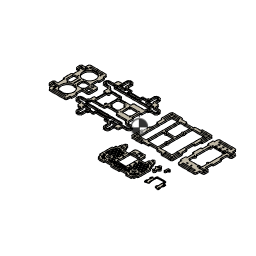
v109 (Autodesk Fusion 360 design; units mm, degrees)
Autodesk Fusion 360 part; units mm, degrees
note: some values were not read from the file. Set by a fixed rule: which sketch regions a step uses.
(part 1 of 3)
sketch "Schizzo1" plane through (0, 0, 0) normal (0, 1, 0) x (1, 0, 0)
  line L0 (-131, 140) -> (-131, 145)
  line L1 (-131, 145) -> (-111, 145)
  line L2 (-111, 140) -> (-131, 140)
  line L3 (-111, 145) -> (-111, 140)
  line L4 (-86, 145) -> (-86, 140)
  line L5 (-86, 140) -> (-71, 140)
  line L6 (-106, 147) -> (-106, 148)
  line L7 (-141, 150) -> (-108, 150)
  arc A0 (-106, 147) -> (-104, 145) centre (-104, 147) ccw
  arc A1 (-106, 148) -> (-108, 150) centre (-108, 148) ccw
  line L8 (25, 10) -> (25, 5)
  line L9 (30, 0) -> (57.5, 0)
  arc A2 (25, 5) -> (30, 0) centre (30, 5) ccw
  arc A3 (-141, 150) -> (-146, 145) centre (-141, 145) ccw
  line L10 (25, 15) -> (20, 15)
  line L11 (20, 35) -> (25, 35)
  line L12 (25, 60) -> (20, 60)
  line L13 (20, 60) -> (20, 75)
  line L14 (25, 10) -> (25, 15)
  line L15 (25, 35) -> (25, 60)
  line L16 (-141, 90) -> (-136, 90)
  line L17 (-136, 90) -> (-136, 75)
  line L18 (-143, 110) -> (-144, 110)
  line L19 (-146, 112) -> (-146, 145)
  arc A4 (-146, 112) -> (-144, 110) centre (-144, 112) ccw
  arc A5 (-141, 108) -> (-143, 110) centre (-143, 108) ccw
  line L20 (-141, 115) -> (-136, 115)
  line L21 (-136, 115) -> (-136, 135)
  line L22 (-136, 135) -> (-141, 135)
  line L23 (-141, 135) -> (-141, 115)
  arc A6 (-108, 0) -> (-106, 2) centre (-108, 2) ccw
  line L24 (-106, 3) -> (-106, 2)
  arc A7 (-104, 5) -> (-106, 3) centre (-104, 3) ccw
  line L25 (-86, 5) -> (-86, 10)
  line L26 (-86, 10) -> (-71, 10)
  line L27 (-136, 60) -> (-136, 75)
  line L28 (-141, 60) -> (-136, 60)
  arc A8 (-143, 40) -> (-141, 42) centre (-143, 42) ccw
  line L29 (-143, 40) -> (-144, 40)
  arc A9 (-144, 40) -> (-146, 38) centre (-144, 38) ccw
  line L30 (-146, 38) -> (-146, 5)
  arc A10 (-146, 5) -> (-141, 0) centre (-141, 5) ccw
  line L31 (-141, 0) -> (-108, 0)
  line L32 (-111, 10) -> (-131, 10)
  line L33 (-131, 10) -> (-131, 5)
  line L34 (-111, 5) -> (-111, 10)
  line L35 (-131, 5) -> (-111, 5)
  line L36 (-141, 15) -> (-141, 35)
  line L37 (-141, 35) -> (-136, 35)
  line L38 (-136, 15) -> (-141, 15)
  line L39 (-136, 35) -> (-136, 15)
  arc A11 (1, 110) -> (-1, 108) centre (1, 108) ccw
  line L40 (1, 110) -> (2, 110)
  arc A12 (2, 110) -> (4, 112) centre (2, 112) ccw
  line L41 (4, 112) -> (4, 145)
  arc A13 (4, 145) -> (-1, 150) centre (-1, 145) ccw
  line L42 (-1, 150) -> (-34, 150)
  arc A14 (-34, 150) -> (-36, 148) centre (-34, 148) ccw
  line L43 (-36, 147) -> (-36, 148)
  arc A15 (-38, 145) -> (-36, 147) centre (-38, 147) ccw
  line L44 (-56, 145) -> (-56, 140)
  line L45 (-56, 140) -> (-71, 140)
  line L46 (-31, 140) -> (-11, 140)
  line L47 (-11, 140) -> (-11, 145)
  line L48 (-31, 145) -> (-31, 140)
  line L49 (-11, 145) -> (-31, 145)
  line L50 (-1, 135) -> (-1, 115)
  line L51 (-1, 115) -> (-6, 115)
  line L52 (-6, 135) -> (-1, 135)
  line L53 (-6, 115) -> (-6, 135)
  line L54 (-1, 90) -> (-6, 90)
  line L55 (-6, 90) -> (-6, 75)
  line L56 (-1, 60) -> (-6, 60)
  line L57 (-6, 60) -> (-6, 75)
  line L58 (-56, 5) -> (-56, 10)
  line L59 (-56, 10) -> (-71, 10)
  arc A16 (-1, 42) -> (1, 40) centre (1, 42) ccw
  line L60 (1, 40) -> (2, 40)
  arc A17 (4, 38) -> (2, 40) centre (2, 38) ccw
  line L61 (4, 38) -> (4, 5)
  arc A18 (-1, 0) -> (4, 5) centre (-1, 5) ccw
  line L62 (-1, 0) -> (-34, 0)
  arc A19 (-36, 2) -> (-34, 0) centre (-34, 2) ccw
  line L63 (-36, 3) -> (-36, 2)
  arc A20 (-36, 3) -> (-38, 5) centre (-38, 3) ccw
  line L64 (-11, 10) -> (-11, 5)
  line L65 (-11, 5) -> (-31, 5)
  line L66 (-31, 10) -> (-11, 10)
  line L67 (-31, 5) -> (-31, 10)
  line L68 (-1, 15) -> (-1, 35)
  line L69 (-1, 35) -> (-6, 35)
  line L70 (-6, 15) -> (-1, 15)
  line L71 (-6, 35) -> (-6, 15)
  line L72 (-231.9997, 2.9999) -> (-231.9997, 2.0006)
  line L73 (-192, 38) -> (-192, 37.0001)
  line L74 (-307, 5) -> (-307, 10)
  line L75 (-197, 60) -> (-202, 60)
  arc A21 (-300, 5) -> (-302, 3) centre (-300, 3) ccw
  arc A22 (-304, 0) -> (-302, 2) centre (-304, 2) ccw
  arc A23 (-197, -0.0001) -> (-192, 4.9999) centre (-197, 4.9999) ccw
  arc A24 (-197, 42) -> (-195, 40) centre (-195, 42) ccw
  arc A25 (-342.0001, 5) -> (-337, 0) centre (-337, 5) ccw
  line L76 (-302, 3) -> (-302, 2)
  line L77 (-195, 40) -> (-194, 40)
  arc A26 (-340, 40) -> (-342, 38) centre (-340, 38) ccw
  arc A27 (-192, 38) -> (-194, 40) centre (-194, 38) ccw
  line L78 (-339, 40) -> (-340, 40)
  line L79 (-202, 60) -> (-202, 75)
  arc A28 (-339, 40) -> (-337, 42) centre (-339, 42) ccw
  arc A29 (-231.9997, 2.9999) -> (-233.9999, 5.0001) centre (-233.9999, 2.9999) ccw
  arc A30 (-231.9997, 2.0006) -> (-229.999, -0.0001) centre (-229.999, 2.0006) ccw
  line L80 (85, 0) -> (57.5, 0)
  arc A31 (85, 0) -> (90, 5) centre (85, 5) ccw
  line L81 (90, 35) -> (90, 60)
  line L82 (90, 60) -> (95, 60)
  line L83 (95, 60) -> (95, 75)
  line L84 (20, 115) -> (25, 115)
  line L85 (25, 115) -> (25, 90)
  line L86 (25, 90) -> (20, 90)
  line L87 (20, 90) -> (20, 75)
  line L88 (25, 140) -> (25, 145)
  line L89 (30, 150) -> (57.5, 150)
  arc A32 (30, 150) -> (25, 145) centre (30, 145) ccw
  line L90 (25, 135) -> (20, 135)
  line L91 (25, 140) -> (25, 135)
  line L92 (57.5, 140) -> (35, 140)
  line L93 (35, 145) -> (35, 140)
  line L94 (57.5, 145) -> (35, 145)
  line L95 (80, 145) -> (80, 140)
  line L96 (80, 140) -> (57.5, 140)
  line L97 (57.5, 145) -> (80, 145)
  arc A33 (90, 145) -> (85, 150) centre (85, 145) ccw
  line L98 (85, 150) -> (57.5, 150)
  line L99 (90, 90) -> (95, 90)
  line L100 (95, 90) -> (95, 75)
  line L101 (-452, 90) -> (-452, 75)
  line L102 (-452, 60) -> (-452, 75)
  line L103 (-452, 115) -> (-457, 115)
  line L104 (-437, 5) -> (-437, 10)
  line L105 (-382, 35) -> (-382, 57.5)
  line L106 (-442, 150) -> (-414.5, 150)
  line L107 (-357, 62.5) -> (-357, 75)
  line L108 (-447, 140) -> (-447, 145)
  line L109 (-377, 115) -> (-382, 115)
  line L110 (-357, 87.5) -> (-357, 75)
  line L111 (-447, 35) -> (-447, 60)
  arc A34 (-442, 150) -> (-447, 145) centre (-442, 145) ccw
  line L112 (-382, 92.5) -> (-362, 92.5)
  line L113 (-382, 140) -> (-382, 135)
  line L114 (-447, 115) -> (-447, 90)
  line L115 (-382, 135) -> (-377, 135)
  line L116 (-382, 140) -> (-382, 145)
  line L117 (-452, 115) -> (-447, 115)
  line L118 (-382, 10) -> (-382, 5)
  line L119 (-392, 5) -> (-392, 10)
  line L120 (-457, 115) -> (-457, 115)
  line L121 (-462, 130) -> (-462, 120)
  arc A35 (-462, 120) -> (-457, 115) centre (-457, 120) ccw
  arc A36 (-457, 135) -> (-462, 130) centre (-457, 130) ccw
  line L122 (-414.5, 5) -> (-437, 5)
  arc A37 (-382, 145) -> (-387, 150) centre (-387, 145) ccw
  line L123 (-447, 10) -> (-447, 5)
  line L124 (-382, 10) -> (-382, 15)
  line L125 (-447, 140) -> (-447, 135)
  line L126 (-382, 115) -> (-382, 92.5)
  line L127 (-387, 0) -> (-414.5, 0)
  line L128 (-377, 35) -> (-382, 35)
  line L129 (-447, 10) -> (-447, 15)
  line L130 (-387, 150) -> (-414.5, 150)
  line L131 (-382, 57.5) -> (-362, 57.5)
  arc A38 (-387, 0) -> (-382, 5) centre (-387, 5) ccw
  line L132 (-414.5, 5) -> (-392, 5)
  line L133 (-442, 0) -> (-414.5, 0)
  line L134 (-382, 15) -> (-377, 15)
  line L135 (-447, 90) -> (-452, 90)
  line L136 (-447, 60) -> (-452, 60)
  arc A39 (-447, 5) -> (-442, 0) centre (-442, 5) ccw
  arc A40 (-357, 87.5) -> (-362, 92.5) centre (-362, 87.5) ccw
  arc A41 (-362, 57.5) -> (-357, 62.5) centre (-362, 62.5) ccw
  circle A42 centre (-252.9, 89.1) radius 1.25
  circle A43 centre (-281.1, 60.9) radius 1.25
  line L137 (-252.9, 84.1) -> (-250.5, 84.1)
  line L138 (-257.9, 89.1) -> (-257.9, 91.5)
  line L139 (-281.1, 65.9) -> (-283.5, 65.9)
  line L140 (-276.1, 60.9) -> (-276.1, 58.5)
  arc A44 (-257.9, 89.1) -> (-252.9, 84.1) centre (-252.9, 89.1) ccw
  arc A45 (-276.1, 60.9) -> (-281.1, 65.9) centre (-281.1, 60.9) ccw
  arc A46 (-248, 81.6) -> (-250.5, 84.1) centre (-250.5, 81.6) ccw
  arc A47 (-257.9, 91.5) -> (-260.4, 94) centre (-260.4, 91.5) ccw
  arc A48 (-286, 68.4) -> (-283.5, 65.9) centre (-283.5, 68.4) ccw
  arc A49 (-276.1, 58.5) -> (-273.6, 56) centre (-273.6, 58.5) ccw
  line L141 (-31, 140) -> (-25, 140)
  line L142 (-337, 42) -> (-337, 57.5)
  line L143 (-300, 5) -> (-286.5, 5)
  line L144 (-247.5, 5.0001) -> (-233.9999, 5.0001)
  circle A50 centre (33, 54) radius 1.5
  circle A51 centre (33, 112) radius 1.5
  circle A52 centre (-115.5198, -118.5231) radius 1.5
  circle A53 centre (-134.2581, -99.7848) radius 1.5
  circle A54 centre (-120.8585, -105.1234) radius 6
  circle A55 centre (-98.9028, -64.4294) radius 1.5
  line L145 (-82.3205, -124) -> (-80, -124)
  line L146 (-85, -121) -> (-85, -122)
  line L147 (-132, -119) -> (-133, -119)
  line L148 (-135, -117) -> (-135, -116)
  line L149 (-130, -61) -> (-130, -62)
  line L150 (-120, -62) -> (-120, -61)
  line L151 (-80, -124) -> (-77.6795, -124)
  line L152 (-75, -114) -> (-79.3301, -116.5)
  line L153 (-79.3301, -116.5) -> (-79.3301, -121.5)
  line L154 (-79.3301, -121.5) -> (-75, -124)
  arc A56 (-85, -121) -> (-87, -119) centre (-87, -121) ccw
  arc A57 (-85, -122) -> (-84.2458, -123.5646) centre (-83, -122) ccw
  arc A58 (-135, -117) -> (-133, -119) centre (-133, -117) ccw
  arc A59 (-135, -116) -> (-135.7542, -114.4354) centre (-137, -116) ccw
  arc A60 (-130.6699, -119.5064) -> (-132, -119) centre (-132, -121) ccw
  arc A61 (-128, -59) -> (-130, -61) centre (-128, -61) ccw
  arc A62 (-120, -61) -> (-122, -59) centre (-122, -61) ccw
  arc A63 (-103.7753, -65.5513) -> (-105.7243, -64) centre (-105.7243, -66) ccw
  line L155 (-75, -114) -> (-79.3301, -116.5)
  line L156 (-79.3301, -116.5) -> (-79.3301, -121.5)
  line L157 (-79.3301, -121.5) -> (-75, -124)
  arc A64 (-120.6699, -117.2162) -> (-122.2488, -116.0352) centre (-122.5016, -118.0192) ccw
  arc A65 (-130.5673, -96.4116) -> (-127.8245, -96.6102) centre (-129.091, -95.0624) ccw
  arc A66 (-112.3453, -112.0894) -> (-112.7588, -113.747) centre (-110.7974, -113.356) ccw
  line L158 (-84.2458, -123.5646) -> (-80.6699, -121.5)
  line L159 (-80.6699, -121.5) -> (-80.6699, -116.5)
  line L160 (-80.6699, -116.5) -> (-85, -114)
  line L161 (-85, -114) -> (-89.3301, -116.5)
  line L162 (-89.3301, -116.5) -> (-89.3301, -119)
  line L163 (-90.6699, -119) -> (-90.6699, -116.5)
  line L164 (-90.6699, -116.5) -> (-95, -114)
  line L165 (-95, -114) -> (-99.3301, -116.5)
  line L166 (-99.3301, -116.5) -> (-99.3301, -119)
  line L167 (-126.72, -114.993) -> (-129.3301, -116.5)
  line L168 (-129.3301, -116.5) -> (-129.3301, -121.5)
  line L169 (-129.3301, -121.5) -> (-125, -124)
  line L170 (-125, -124) -> (-120.6699, -121.5)
  line L171 (-120.6699, -121.5) -> (-120.6699, -117.2162)
  line L172 (-130.6699, -116.5) -> (-135, -114)
  line L173 (-80, -115.3397) -> (-75.6699, -112.8397)
  line L174 (-75.6699, -112.8397) -> (-75.6699, -107.8397)
  line L175 (-75.6699, -107.8397) -> (-77.9904, -106.5)
  line L176 (-82.0096, -106.5) -> (-84.3301, -107.8398)
  line L177 (-84.3301, -107.8398) -> (-84.3301, -112.8398)
  line L178 (-84.3301, -112.8398) -> (-80, -115.3397)
  line L179 (-85.6699, -112.8397) -> (-85.6699, -107.8397)
  line L180 (-85.6699, -107.8397) -> (-87.9002, -106.5521)
  line L181 (-92.1651, -106.5898) -> (-94.3301, -107.8398)
  line L182 (-94.3301, -107.8398) -> (-94.3301, -112.8398)
  line L183 (-94.3301, -112.8398) -> (-90, -115.3397)
  line L184 (-90, -115.3397) -> (-85.6699, -112.8397)
  line L185 (-75.6699, -112.8397) -> (-75.6699, -107.8397)
  line L186 (-75.6699, -107.8397) -> (-77.9904, -106.5)
  line L187 (-82.0096, -106.5) -> (-84.3301, -107.8398)
  line L188 (-84.3301, -107.8398) -> (-84.3301, -112.8398)
  line L189 (-84.3301, -112.8398) -> (-80, -115.3397)
  line L190 (-80, -115.3397) -> (-75.6699, -112.8397)
  line L191 (-105.6699, -107.8397) -> (-109.8624, -105.4192)
  line L192 (-112.7588, -113.747) -> (-110, -115.3397)
  line L193 (-110, -115.3397) -> (-105.6699, -112.8397)
  line L194 (-105.6699, -112.8397) -> (-105.6699, -107.8397)
  line L195 (-100, -115.3397) -> (-95.6699, -112.8397)
  line L196 (-95.6699, -112.8397) -> (-95.6699, -107.8397)
  line L197 (-95.6699, -107.8397) -> (-100, -105.3397)
  line L198 (-100, -105.3397) -> (-104.3301, -107.8398)
  line L199 (-104.3301, -112.8398) -> (-100, -115.3397)
  line L200 (-104.3301, -107.8398) -> (-104.3301, -112.8398)
  line L201 (-130, -115.3397) -> (-127.4968, -113.8945)
  line L202 (-131.7929, -106.3749) -> (-134.3301, -107.8398)
  line L203 (-134.3301, -112.8398) -> (-130, -115.3397)
  line L204 (-134.3301, -107.8398) -> (-134.3301, -112.8398)
  line L205 (-80, -122.6603) -> (-82.3205, -124)
  line L206 (-77.6795, -124) -> (-80, -122.6603)
  line L207 (-100.6699, -99.1795) -> (-105, -96.6795)
  line L208 (-105, -96.6795) -> (-109.3301, -99.1795)
  line L209 (-109.3301, -99.1795) -> (-109.3301, -104.1795)
  line L210 (-109.3301, -104.1795) -> (-105, -106.6795)
  line L211 (-100.6699, -104.1795) -> (-100.6699, -99.1795)
  line L212 (-105, -106.6795) -> (-100.6699, -104.1795)
  line L213 (-135, -106.6795) -> (-132.4803, -105.2248)
  line L214 (-139.3301, -103) -> (-139.3301, -104.1795)
  line L215 (-139.3301, -104.1795) -> (-135, -106.6795)
  line L216 (-105.6699, -90.5192) -> (-110, -88.0192)
  line L217 (-110, -88.0192) -> (-114.3301, -90.5192)
  line L218 (-114.3301, -90.5192) -> (-114.3301, -95.5192)
  line L219 (-114.3301, -95.5192) -> (-110, -98.0192)
  line L220 (-110, -98.0192) -> (-105.6699, -95.5192)
  line L221 (-105.6699, -95.5192) -> (-105.6699, -90.5192)
  line L222 (-125.6699, -90.5192) -> (-130, -88.0192)
  line L223 (-130, -88.0192) -> (-134.3301, -90.5192)
  line L224 (-134.3301, -90.5192) -> (-134.3301, -94.7853)
  line L225 (-125.6699, -95.2315) -> (-125.6699, -90.5192)
  line L226 (-115.6699, -95.424) -> (-115.6699, -90.5192)
  line L227 (-115.6699, -90.5192) -> (-120, -88.0192)
  line L228 (-120, -88.0192) -> (-124.3301, -90.5192)
  line L229 (-124.3301, -90.5192) -> (-124.3301, -94.6856)
  line L230 (-140, -98.0192) -> (-138.5149, -97.1618)
  line L231 (-135.6699, -94.9882) -> (-135.6699, -90.5192)
  line L232 (-135.6699, -90.5192) -> (-140, -88.0192)
  line L233 (-100.6699, -81.859) -> (-105, -79.359)
  line L234 (-105, -79.359) -> (-109.3301, -81.859)
  line L235 (-109.3301, -81.859) -> (-109.3301, -86.859)
  line L236 (-109.3301, -86.859) -> (-105, -89.359)
  line L237 (-100.6699, -86.859) -> (-100.6699, -81.859)
  line L238 (-105, -89.359) -> (-100.6699, -86.859)
  line L239 (-110.6699, -86.859) -> (-110.6699, -81.859)
  line L240 (-110.6699, -81.859) -> (-115, -79.359)
  line L241 (-115, -79.359) -> (-119.3301, -81.859)
  line L242 (-119.3301, -81.859) -> (-119.3301, -86.859)
  line L243 (-119.3301, -86.859) -> (-115, -89.359)
  line L244 (-115, -89.359) -> (-110.6699, -86.859)
  line L245 (-120.6699, -81.859) -> (-125, -79.359)
  line L246 (-125, -79.359) -> (-129.3301, -81.859)
  line L247 (-129.3301, -81.859) -> (-129.3301, -86.859)
  line L248 (-129.3301, -86.859) -> (-125, -89.359)
  line L249 (-120.6699, -86.859) -> (-120.6699, -81.859)
  line L250 (-125, -89.359) -> (-120.6699, -86.859)
  line L251 (-130.6699, -86.859) -> (-130.6699, -81.859)
  line L252 (-130.6699, -81.859) -> (-135, -79.359)
  line L253 (-135, -79.359) -> (-139.3301, -81.859)
  line L254 (-139.3301, -81.859) -> (-139.3301, -86.859)
  line L255 (-139.3301, -86.859) -> (-135, -89.359)
  line L256 (-135, -89.359) -> (-130.6699, -86.859)
  line L257 (-134.3301, -73.1987) -> (-134.3301, -78.1987)
  line L258 (-134.3301, -78.1987) -> (-130, -80.6987)
  line L259 (-130, -80.6987) -> (-125.6699, -78.1987)
  line L260 (-125.6699, -78.1987) -> (-125.6699, -73.1987)
  line L261 (-125.6699, -73.1987) -> (-130, -70.6987)
  line L262 (-130, -70.6987) -> (-134.3301, -73.1987)
  line L263 (-124.3301, -78.1987) -> (-120, -80.6987)
  line L264 (-120, -80.6987) -> (-115.6699, -78.1987)
  line L265 (-115.6699, -78.1987) -> (-115.6699, -73.1987)
  line L266 (-115.6699, -73.1987) -> (-120, -70.6987)
  line L267 (-124.3301, -73.1987) -> (-124.3301, -78.1987)
  line L268 (-120, -70.6987) -> (-124.3301, -73.1987)
  line L269 (-114.3301, -78.1987) -> (-110, -80.6987)
  line L270 (-110, -80.6987) -> (-105.6699, -78.1987)
  line L271 (-105.6699, -78.1987) -> (-105.6699, -73.1987)
  line L272 (-105.6699, -73.1987) -> (-110, -70.6987)
  line L273 (-114.3301, -73.1987) -> (-114.3301, -78.1987)
  line L274 (-110, -70.6987) -> (-114.3301, -73.1987)
  line L275 (-108.3975, -64) -> (-109.3301, -64.5385)
  line L276 (-109.3301, -64.5385) -> (-109.3301, -69.5385)
  line L277 (-109.3301, -69.5385) -> (-105, -72.0385)
  line L278 (-105, -72.0385) -> (-100.6699, -69.5385)
  line L279 (-100.6699, -69.5385) -> (-100.6699, -69.1067)
  line L280 (-118.3454, -63.9699) -> (-119.3301, -64.5385)
  line L281 (-119.3301, -64.5385) -> (-119.3301, -69.5385)
  line L282 (-119.3301, -69.5385) -> (-115, -72.0385)
  line L283 (-115, -72.0385) -> (-110.6699, -69.5385)
  line L284 (-110.6699, -64.5385) -> (-111.6025, -64)
  line L285 (-110.6699, -69.5385) -> (-110.6699, -64.5385)
  line L286 (-125, -62.0385) -> (-129.3301, -64.5385)
  line L287 (-129.3301, -64.5385) -> (-129.3301, -69.5385)
  line L288 (-129.3301, -69.5385) -> (-125, -72.0385)
  line L289 (-125, -72.0385) -> (-120.6699, -69.5385)
  line L290 (-120.6699, -64.5385) -> (-125, -62.0385)
  line L291 (-120.6699, -69.5385) -> (-120.6699, -64.5385)
  line L292 (-120, -63.3782) -> (-119.6271, -63.1629)
  line L293 (-124.3301, -59) -> (-124.3301, -60.8782)
  line L294 (-124.3301, -60.8782) -> (-120, -63.3782)
  line L295 (-130.3729, -63.163) -> (-130, -63.3782)
  line L296 (-130, -63.3782) -> (-125.6699, -60.8782)
  line L297 (-125.6699, -60.8782) -> (-125.6699, -59)
  line L298 (-87, -119) -> (-89.3301, -119)
  line L299 (-90.6699, -119) -> (-99.3301, -119)
  arc A67 (-112.3453, -112.0894) -> (-109.8624, -105.4192) centre (-120.8585, -105.1234) ccw
  arc A68 (-115.6699, -95.424) -> (-124.3301, -94.6856) centre (-120.8585, -105.1234) ccw
  arc A69 (-125.6699, -95.2315) -> (-127.8245, -96.6102) centre (-120.8585, -105.1234) ccw
  arc A70 (-130.5673, -96.4116) -> (-134.3301, -94.7853) centre (-134.2581, -99.7848) ccw
  arc A71 (-135.6699, -94.9882) -> (-138.5149, -97.1618) centre (-134.2581, -99.7848) ccw
  arc A72 (-138.0873, -103) -> (-133.8982, -104.7718) centre (-134.2581, -99.7848) ccw
  arc A73 (-131.7702, -106.5138) -> (-131.7929, -106.3749) centre (-133.7542, -106.7666) ccw
  arc A74 (-132.4803, -105.2248) -> (-133.8982, -104.7718) centre (-133.7542, -106.7666) ccw
  line L300 (-140, -88.0192) -> (-140, -98.0192)
  arc A75 (-130.3729, -63.163) -> (-130, -62) centre (-132, -62) ccw
  line L301 (-122, -59) -> (-124.3301, -59)
  line L302 (-125.6699, -59) -> (-128, -59)
  arc A76 (-120, -62) -> (-119.6271, -63.1629) centre (-118, -62) ccw
  arc A77 (-118.3454, -63.9699) -> (-118, -64) centre (-118, -62) ccw
  line L303 (-118, -64) -> (-111.6025, -64)
  line L304 (-108.3975, -64) -> (-105.7243, -64)
  arc A78 (-103.7753, -65.5513) -> (-100.6699, -69.1067) centre (-98.9028, -64.4294) ccw
  line L305 (-135, -114) -> (-135.7542, -114.4354)
  line L306 (-130.6699, -116.5) -> (-130.6699, -119.5064)
  line L307 (-60, -124) -> (-35, -124)
  line L308 (-60, -124) -> (-60, -129)
  line L309 (-35, -124) -> (-35, -129)
  line L310 (-15, -129) -> (-15, -124)
  line L311 (-35, -129) -> (-15, -129)
  arc A79 (-55.5, -39) -> (-60.5, -34) centre (-60.5, -39) ccw
  line L312 (-55.5, -59) -> (-55.5, -39)
  line L313 (-35, -59) -> (-55.5, -59)
  line L314 (-35, -59) -> (-35, -54)
  line L315 (-30, -54) -> (-20, -54)
  line L316 (-15, -54) -> (-15, -59)
  line L317 (-10, -59) -> (-15, -59)
  line L318 (-10, -69) -> (-5, -69)
  line L319 (-5, -69) -> (-5, -114)
  line L320 (-15, -124) -> (-10, -124)
  line L321 (-5, -114) -> (-10, -114)
  circle A80 centre (-29.1416, -105.1234) radius 6
  circle A81 centre (-34.4802, -118.5231) radius 1.5
  circle A82 centre (-15.7419, -99.7848) radius 1.5
  line L322 (-75, -114) -> (-75, -114)
  circle A83 centre (-51.0972, -64.4294) radius 1.5
  circle A84 centre (82, 54) radius 1.5
  circle A85 centre (82, 112) radius 1.5
  circle A86 centre (-91, 75) radius 1.5
  circle A87 centre (-59, 45) radius 1.5
  arc A88 (-131, 18) -> (-128, 15) centre (-128, 18) ccw
  arc A89 (-61.5, 69.5) -> (-64.5, 72.5) centre (-64.5, 69.5) ccw
  line L323 (-11, 17.5) -> (-11, 75)
  line L324 (-13.9289, 15) -> (-13.5, 15)
  arc A90 (-56.5, 17.5) -> (-54, 15) centre (-54, 17.5) ccw
  arc A91 (-13.5, 15) -> (-11, 17.5) centre (-13.5, 17.5) ccw
  circle A92 centre (-392, 15) radius 1.5
  circle A93 centre (-432, 55) radius 1.5
  line L325 (-260.4, 94) -> (-278, 94)
  line L326 (-286, 86) -> (-286, 68.4)
  line L327 (-273.6, 56) -> (-256, 56)
  line L328 (-248, 64) -> (-248, 81.6)
  arc A94 (-278, 94) -> (-286, 86) centre (-278, 86) ccw
  arc A95 (-256, 56) -> (-248, 64) centre (-256, 64) ccw
  arc A96 (-64.5, 15) -> (-61.5, 18) centre (-64.5, 18) ccw
  arc A97 (-128, 135) -> (-131, 132) centre (-128, 132) ccw
  line L329 (-100, 18) -> (-100, 69.5)
  line L330 (-105, 18) -> (-105, 132)
  line L331 (-64.5, 15) -> (-97, 15)
  line L332 (-131, 18) -> (-131, 132)
  arc A98 (-97, 72.5) -> (-100, 69.5) centre (-97, 69.5) ccw
  arc A99 (-100, 18) -> (-97, 15) centre (-97, 18) ccw
  arc A100 (-108, 15) -> (-105, 18) centre (-108, 18) ccw
  arc A101 (-105, 132) -> (-108, 135) centre (-108, 132) ccw
  circle A102 centre (-292, 55) radius 1.5
  circle A103 centre (-322, 95) radius 1.5
  line L333 (-377, 135) -> (-377, 115)
  line L334 (-377, 35) -> (-377, 15)
  line L335 (-326, 91) -> (-326, 50)
  line L336 (-322, 46) -> (-294, 46)
  line L337 (-292, 48) -> (-292, 49.3431)
  line L338 (-322, 100.6569) -> (-322, 102)
  line L339 (-288, 59) -> (-288, 100)
  line L340 (-320, 104) -> (-292, 104)
  arc A104 (-324.4, 91.8) -> (-320.6667, 98.7712) centre (-322, 95) ccw
  arc A105 (-289.6, 58.2) -> (-293.3333, 51.2288) centre (-292, 55) ccw
  arc A106 (-326, 50) -> (-322, 46) centre (-322, 50) ccw
  arc A107 (-288, 100) -> (-292, 104) centre (-292, 100) ccw
  arc A108 (-294, 46) -> (-292, 48) centre (-294, 48) ccw
  arc A109 (-320, 104) -> (-322, 102) centre (-320, 102) ccw
  arc A110 (-289.6, 58.2) -> (-288, 59) centre (-289, 59) ccw
  arc A111 (-324.4, 91.8) -> (-326, 91) centre (-325, 91) ccw
  arc A112 (-292, 49.3431) -> (-293.3333, 51.2288) centre (-294, 49.3431) ccw
  arc A113 (-322, 100.6569) -> (-320.6667, 98.7712) centre (-320, 100.6569) ccw
  line L341 (-62.5, -38.44) -> (-76.5, -38.44)
  line L342 (-76.5, -38.44) -> (-76.5, -52.44)
  line L343 (-76.5, -52.44) -> (-62.5, -52.44)
  line L344 (-62.5, -52.44) -> (-62.5, -38.44)
  line L345 (-361.44, 62.5) -> (-375.44, 62.5)
  line L346 (-375.44, 62.5) -> (-375.44, 76.5)
  line L347 (-375.44, 76.5) -> (-361.44, 76.5)
  line L348 (-361.44, 76.5) -> (-361.44, 62.5)
  line L349 (20, 15) -> (20, 35)
  line L350 (20, 115) -> (20, 135)
  line L351 (-366, 23.0002) -> (-366, 27.0001)
  line L352 (-342, 38) -> (-342, 37.0001)
  line L353 (-342, 13.0001) -> (-342.0001, 5)
  arc A114 (-344, 35.0001) -> (-342, 37.0001) centre (-344, 37.0001) ccw
  arc A115 (-342, 13.0001) -> (-344, 15.0001) centre (-344, 13.0001) ccw
  arc A116 (-358, 35.0001) -> (-366, 27.0001) centre (-358, 27.0001) ccw
  arc A117 (-366, 23.0002) -> (-358, 15.0002) centre (-358, 23.0002) ccw
  line L354 (-307, -2) -> (-307, -15.9102)
  line L355 (-315, -23.9102) -> (-319, -23.9102)
  line L356 (-327, -15.9102) -> (-327, -2)
  line L357 (-337, 0) -> (-329, 0)
  line L358 (-305, 0) -> (-304, 0)
  arc A118 (-327, -2) -> (-329, 0) centre (-329, -2) ccw
  arc A119 (-305, 0) -> (-307, -2) centre (-305, -2) ccw
  arc A120 (-327, -15.9102) -> (-319, -23.9102) centre (-319, -15.9102) ccw
  arc A121 (-315, -23.9102) -> (-307, -15.9102) centre (-315, -15.9102) ccw
  line L359 (-227, -2.0001) -> (-227, -15.9189)
  arc A122 (-227, -15.9189) -> (-219, -23.9102) centre (-219, -15.9102) ccw
  line L360 (-219, -23.9102) -> (-215, -23.9102)
  arc A123 (-215, -23.9102) -> (-207, -15.9246) centre (-215, -15.9102) ccw
  line L361 (-207, -15.9246) -> (-207, -2.0001)
  arc A124 (-205, -0.0001) -> (-207, -2.0001) centre (-205, -2.0001) ccw
  arc A125 (-227, -2.0001) -> (-229, -0.0001) centre (-229, -2.0001) ccw
  line L362 (-197, -0.0001) -> (-205, -0.0001)
  line L363 (-229, -0.0001) -> (-229.999, -0.0001)
  arc A126 (-190, 15.0001) -> (-192, 13.0001) centre (-190, 13.0001) ccw
  arc A127 (-175.9914, 15.0002) -> (-168, 23.0002) centre (-176, 23.0002) ccw
  line L364 (-168, 23.0002) -> (-168, 27.0001)
  arc A128 (-168, 27.0001) -> (-176, 35.0001) centre (-176, 27.0001) ccw
  arc A129 (-192, 37.0001) -> (-190, 35.0001) centre (-190, 37.0001) ccw
  line L365 (-192, 4.9999) -> (-192, 13.0001)
  line L366 (33, 35) -> (33, 46.5838)
  line L367 (33, 61.4162) -> (33, 104.5838)
  arc A130 (34.875, 49.3649) -> (34.875, 58.6351) centre (33, 54) ccw
  arc A131 (33, 35) -> (38, 30) centre (38, 35) ccw
  arc A132 (34.875, 49.3649) -> (33, 46.5838) centre (36, 46.5838) ccw
  arc A133 (33, 61.4162) -> (34.875, 58.6351) centre (36, 61.4162) ccw
  arc A134 (34.875, 107.3649) -> (33, 104.5838) centre (36, 104.5838) ccw
  line L368 (82, 35) -> (82, 46.5838)
  arc A135 (82, 46.5838) -> (80.125, 49.3649) centre (79, 46.5838) ccw
  arc A136 (80.125, 58.6351) -> (80.125, 49.3649) centre (82, 54) ccw
  arc A137 (80.125, 58.6351) -> (82, 61.4162) centre (79, 61.4162) ccw
  line L369 (82, 61.4162) -> (82, 104.5838)
  arc A138 (82, 104.5838) -> (80.125, 107.3649) centre (79, 104.5838) ccw
  line L370 (33, 118) -> (33, 117.9161)
  line L371 (82, 118) -> (82, 117.9161)
  arc A139 (34.875, 107.3649) -> (33.8333, 116.9301) centre (33, 112) ccw
  arc A140 (81.1667, 116.9301) -> (80.125, 107.3649) centre (82, 112) ccw
  arc A141 (33, 117.9161) -> (33.8333, 116.9301) centre (34, 117.9161) ccw
  arc A142 (34, 119) -> (33, 118) centre (34, 118) ccw
  arc A143 (81.1667, 116.9301) -> (82, 117.9161) centre (81, 117.9161) ccw
  arc A144 (82, 118) -> (81, 119) centre (81, 118) ccw
  line L372 (-416, 62.5) -> (-416, 62.5)
  line L373 (-417.5, 63.5) -> (-417.5, 86.5)
  line L374 (-416, 87.5) -> (-416, 87.5)
  line L375 (-415.5, 86.5) -> (-415.5, 63.5)
  arc A145 (-417.5, 63.5) -> (-416.5, 62.5) centre (-416.5, 63.5) ccw
  arc A146 (-416.5, 62.5) -> (-415.5, 63.5) centre (-416.5, 63.5) ccw
  arc A147 (-415.5, 86.5) -> (-416.5, 87.5) centre (-416.5, 86.5) ccw
  arc A148 (-416.5, 87.5) -> (-417.5, 86.5) centre (-416.5, 86.5) ccw
  arc A149 (-131.7702, -106.5138) -> (-127.4968, -113.8945) centre (-120.8585, -105.1234) ccw
  arc A150 (-125.7732, -114.9644) -> (-122.2488, -116.0352) centre (-120.8585, -105.1234) ccw
  line L376 (-109.3301, -116.5) -> (-109.3301, -119)
  line L377 (-105, -114) -> (-109.3301, -116.5)
  line L378 (-100.6699, -116.5) -> (-105, -114)
  line L379 (-100.6699, -119) -> (-100.6699, -116.5)
  line L380 (-100.6699, -119) -> (-109.3301, -119)
  line L381 (-10, -98.0192) -> (-11.4851, -97.1618)
  line L382 (-70, -124) -> (-72.3205, -124)
  line L383 (-37.2412, -113.747) -> (-40, -115.3397)
  line L384 (-45, -96.6795) -> (-40.6699, -99.1795)
  arc A151 (-63, -119) -> (-65, -121) centre (-63, -121) ccw
  line L385 (-14.3301, -78.1987) -> (-14.3301, -73.4936)
  line L386 (-10, -105.3398) -> (-10, -107)
  line L387 (-35, -79.359) -> (-30.6699, -81.859)
  line L388 (-35.6699, -90.5192) -> (-35.6699, -95.5192)
  line L389 (-50, -115.3397) -> (-54.3301, -112.8397)
  line L390 (-64.3301, -112.8397) -> (-64.3301, -107.8397)
  arc A152 (-27.7512, -116.0352) -> (-29.3301, -117.2162) centre (-27.4984, -118.0192) ccw
  line L391 (-34.3301, -95.424) -> (-34.3301, -90.5192)
  line L392 (-55, -114) -> (-50.6699, -116.5)
  arc A153 (-22.5032, -113.8945) -> (-18.2298, -106.5138) centre (-29.1416, -105.1234) ccw
  arc A154 (-25.6699, -94.6856) -> (-34.3301, -95.424) centre (-29.1416, -105.1234) ccw
  line L393 (-25.6699, -90.5192) -> (-25.6699, -94.6856)
  line L394 (-45, -114) -> (-40.6699, -116.5)
  line L395 (-40.6699, -104.1795) -> (-45, -106.6795)
  line L396 (-59.3301, -119) -> (-59.3301, -116.5)
  line L397 (-44.3301, -112.8397) -> (-44.3301, -107.8397)
  line L398 (-63, -119) -> (-60.6699, -119)
  line L399 (-55.6699, -112.8398) -> (-60, -115.3397)
  arc A155 (-22.1755, -96.6102) -> (-19.4327, -96.4116) centre (-20.909, -95.0624) ccw
  line L400 (-74.3301, -112.8397) -> (-74.3301, -107.8397)
  line L401 (-65, -114) -> (-60.6699, -116.5)
  line L402 (-24.3301, -78.1987) -> (-24.3301, -73.1987)
  line L403 (-15, -72.0385) -> (-19.3301, -69.5385)
  line L404 (-60, -115.3397) -> (-64.3301, -112.8397)
  line L405 (-40.6699, -116.5) -> (-40.6699, -119)
  line L406 (-44.3301, -95.5192) -> (-44.3301, -90.5192)
  line L407 (-25, -79.359) -> (-20.6699, -81.859)
  line L408 (-44.3301, -90.5192) -> (-40, -88.0192)
  line L409 (-59.3301, -119) -> (-50.6699, -119)
  line L410 (-65.7542, -123.5646) -> (-69.3301, -121.5)
  line L411 (-20, -70.6987) -> (-15.6699, -73.1987)
  line L412 (-50.6699, -116.5) -> (-50.6699, -119)
  line L413 (-29.3301, -81.859) -> (-25, -79.359)
  line L414 (-60.6699, -116.5) -> (-60.6699, -119)
  line L415 (-70, -115.3397) -> (-74.3301, -112.8397)
  arc A156 (-16.1019, -104.7718) -> (-11.9128, -103) centre (-15.7419, -99.7848) ccw
  line L416 (-49.3301, -104.1795) -> (-49.3301, -99.1795)
  line L417 (-20.6699, -69.5385) -> (-25, -72.0385)
  line L418 (-25, -72.0385) -> (-29.3301, -69.5385)
  line L419 (-25, -124) -> (-29.3301, -121.5)
  line L420 (-55.6699, -107.8398) -> (-55.6699, -112.8398)
  line L421 (-41.6026, -64) -> (-40.6699, -64.5385)
  line L422 (-15.6699, -107.8398) -> (-15.6699, -112.8398)
  line L423 (-39.3301, -64.5385) -> (-38.3975, -64)
  line L424 (-49.3301, -99.1795) -> (-45, -96.6795)
  line L425 (-49.3301, -119) -> (-40.6699, -119)
  line L426 (-30.6699, -69.5385) -> (-35, -72.0385)
  line L427 (-65.6699, -107.8398) -> (-65.6699, -112.8398)
  line L428 (-65.6699, -107.8398) -> (-65.6699, -112.8398)
  line L429 (-39.3301, -81.859) -> (-35, -79.359)
  line L430 (-35, -72.0385) -> (-39.3301, -69.5385)
  line L431 (-14.9997, -72.0383) -> (-15, -72.0385)
  line L432 (-40.6699, -64.5385) -> (-40.6699, -69.5385)
  line L433 (-45, -106.6795) -> (-49.3301, -104.1795)
  line L434 (-39.3301, -69.5385) -> (-39.3301, -64.5385)
  line L435 (-45.6699, -112.8398) -> (-50, -115.3397)
  line L436 (-74.3301, -112.8397) -> (-74.3301, -107.8397)
  arc A157 (-27.7512, -116.0352) -> (-23.759, -114.7165) centre (-29.1416, -105.1234) ccw
  line L437 (-54.3301, -112.8397) -> (-54.3301, -107.8397)
  line L438 (-41.6026, -64) -> (-44.2757, -64)
  line L439 (-14.3301, -109.5064) -> (-14.3301, -107.8397)
  arc A158 (-49.3301, -69.1067) -> (-46.2247, -65.5513) centre (-51.0972, -64.4294) ccw
  line L440 (-40, -70.6987) -> (-35.6699, -73.1987)
  line L441 (-50, -105.3397) -> (-45.6699, -107.8398)
  line L442 (-40.6699, -99.1795) -> (-40.6699, -104.1795)
  arc A159 (-44.2757, -64) -> (-46.2247, -65.5513) centre (-44.2757, -66) ccw
  line L443 (-67.9904, -106.5) -> (-65.6699, -107.8398)
  line L444 (-10.6699, -86.859) -> (-15, -89.359)
  line L445 (-54.3301, -107.8397) -> (-50, -105.3397)
  line L446 (-30.6699, -86.859) -> (-35, -89.359)
  line L447 (-10.6699, -104.1795) -> (-15, -106.6795)
  arc A160 (-22.1755, -96.6102) -> (-24.3301, -95.2315) centre (-29.1416, -105.1234) ccw
  line L448 (-10, -80.6987) -> (-14.3301, -78.1987)
  line L449 (-25.6699, -78.1987) -> (-30, -80.6987)
  line L450 (-30, -63.3782) -> (-30.3729, -63.1629)
  line L451 (-70.6699, -116.5) -> (-70.6699, -121.5)
  line L452 (-19.6271, -63.163) -> (-20, -63.3782)
  line L453 (-49.3301, -86.859) -> (-49.3301, -81.859)
  line L454 (-49.3301, -81.859) -> (-45, -79.359)
  line L455 (-15.6699, -78.1987) -> (-20, -80.6987)
  arc A161 (-16.1019, -104.7718) -> (-17.5197, -105.2248) centre (-16.2458, -106.7666) ccw
  line L456 (-10.0103, -75.7973) -> (-10, -80.6987)
  line L457 (-29.3301, -69.5385) -> (-29.3301, -64.5385)
  line L458 (-14.3301, -107.8397) -> (-10, -105.3397)
  line L459 (-69.3301, -116.5) -> (-65, -114)
  line L460 (-40, -80.6987) -> (-44.3301, -78.1987)
  line L461 (-23.759, -114.7165) -> (-20.6699, -116.5)
  line L462 (-40.6699, -81.859) -> (-40.6699, -86.859)
  line L463 (-14.3301, -90.5192) -> (-10, -88.0192)
  line L464 (-75, -114) -> (-70.6699, -116.5)
  line L465 (-29.3301, -121.5) -> (-29.3301, -117.2162)
  line L466 (-75, -114) -> (-75, -114)
  arc A162 (-20, -61) -> (-22, -59) centre (-22, -61) ccw
  line L467 (-70.6699, -121.5) -> (-75, -124)
  line L468 (-20, -115.3397) -> (-22.5032, -113.8945)
  arc A163 (-18, -119) -> (-19.3301, -119.5064) centre (-18, -121) ccw
  arc A164 (-30.3729, -63.1629) -> (-30, -62) centre (-32, -62) ccw
  line L469 (-34.3301, -73.1987) -> (-30, -70.6987)
  line L470 (-24.3301, -60.8782) -> (-24.3301, -59)
  line L471 (-15.6699, -73.1987) -> (-15.6699, -78.1987)
  line L472 (-15, -106.6795) -> (-17.5197, -105.2248)
  line L473 (-65, -121) -> (-65, -122)
  arc A165 (-15, -66) -> (-17, -64) centre (-17, -66) ccw
  line L474 (-45, -79.359) -> (-40.6699, -81.859)
  line L475 (-39.3301, -86.859) -> (-39.3301, -81.859)
  line L476 (-24.3301, -95.2315) -> (-24.3301, -90.5192)
  line L477 (-10, -88.0192) -> (-10, -98.0192)
  line L478 (-20, -63.3782) -> (-24.3301, -60.8782)
  line L479 (-15, -79.359) -> (-10.6699, -81.859)
  line L480 (-70.6699, -116.5) -> (-70.6699, -121.5)
  line L481 (-44.3301, -73.1987) -> (-40, -70.6987)
  line L482 (-15, -67) -> (-15, -66)
  line L483 (-14.3301, -94.9882) -> (-14.3301, -90.5192)
  line L484 (-18, -119) -> (-17, -119)
  line L485 (-19.3301, -116.5) -> (-15, -114)
  line L486 (-10.6699, -81.859) -> (-10.6699, -86.859)
  line L487 (-25.6699, -73.1987) -> (-25.6699, -78.1987)
  arc A166 (-15.6699, -94.7853) -> (-19.4327, -96.4116) centre (-15.7419, -99.7848) ccw
  line L488 (-31.6546, -63.9699) -> (-30.6699, -64.5385)
  line L489 (-15.6699, -112.8398) -> (-20, -115.3397)
  arc A167 (-11.4851, -97.1618) -> (-14.3301, -94.9882) centre (-15.7419, -99.7848) ccw
  line L490 (-49.3301, -69.5385) -> (-49.3301, -69.1067)
  line L491 (-29.3301, -86.859) -> (-29.3301, -81.859)
  line L492 (-59.3301, -116.5) -> (-55, -114)
  line L493 (-34.3301, -90.5192) -> (-30, -88.0192)
  line L494 (-69.3301, -121.5) -> (-69.3301, -116.5)
  line L495 (-67.6795, -124) -> (-70, -124)
  line L496 (-49.3301, -119) -> (-49.3301, -116.5)
  line L497 (-45, -72.0385) -> (-49.3301, -69.5385)
  line L498 (-24.3301, -90.5192) -> (-20, -88.0192)
  line L499 (-35.6699, -95.5192) -> (-40, -98.0192)
  line L500 (-24.3301, -73.1987) -> (-20, -70.6987)
  line L501 (-30, -80.6987) -> (-34.3301, -78.1987)
  line L502 (-20, -80.6987) -> (-24.3301, -78.1987)
  line L503 (-30, -88.0192) -> (-25.6699, -90.5192)
  line L504 (-18.2071, -106.3749) -> (-15.6699, -107.8398)
  arc A168 (-37.2412, -113.747) -> (-37.6548, -112.0894) centre (-39.2026, -113.356) ccw
  line L505 (-40, -88.0192) -> (-35.6699, -90.5192)
  line L506 (-19.3301, -81.859) -> (-15, -79.359)
  line L507 (-28, -59) -> (-25.6699, -59)
  line L508 (-45.6699, -107.8398) -> (-45.6699, -112.8398)
  line L509 (-65.6699, -112.8398) -> (-70, -115.3397)
  line L510 (-20, -88.0192) -> (-15.6699, -90.5192)
  arc A169 (-18.2071, -106.3749) -> (-18.2298, -106.5138) centre (-16.2458, -106.7666) ccw
  line L511 (-19.3301, -86.859) -> (-19.3301, -81.859)
  line L512 (-40, -98.0192) -> (-44.3301, -95.5192)
  line L513 (-34.3301, -78.1987) -> (-34.3301, -73.1987)
  line L514 (-44.3301, -78.1987) -> (-44.3301, -73.1987)
  line L515 (-70, -115.3397) -> (-74.3301, -112.8397)
  line L516 (-30.6699, -81.859) -> (-30.6699, -86.859)
  line L517 (-20.6699, -81.859) -> (-20.6699, -86.859)
  line L518 (-15, -117) -> (-15, -116)
  arc A170 (-65.7542, -123.5646) -> (-65, -122) centre (-67, -122) ccw
  line L519 (-30, -70.6987) -> (-25.6699, -73.1987)
  line L520 (-44.3301, -107.8397) -> (-40.1376, -105.4192)
  line L521 (-72.3205, -124) -> (-70, -122.6603)
  line L522 (-10.6699, -103) -> (-10.6699, -104.1795)
  arc A171 (-40.1376, -105.4192) -> (-37.6548, -112.0894) centre (-29.1416, -105.1234) ccw
  line L523 (-40, -115.3397) -> (-44.3301, -112.8397)
  line L524 (-40.6699, -69.5385) -> (-45, -72.0385)
  line L525 (-15.6699, -90.5192) -> (-15.6699, -94.7853)
  line L526 (-35.6699, -73.1987) -> (-35.6699, -78.1987)
  line L527 (-67.9904, -106.5) -> (-65.6699, -107.8398)
  line L528 (-74.3301, -107.8397) -> (-72.0096, -106.5)
  line L529 (-74.3301, -107.8397) -> (-72.0096, -106.5)
  line L530 (-40.6699, -86.859) -> (-45, -89.359)
  line L531 (-20.6699, -86.859) -> (-25, -89.359)
  line L532 (-15, -89.359) -> (-19.3301, -86.859)
  line L533 (-35, -89.359) -> (-39.3301, -86.859)
  line L534 (-49.3301, -116.5) -> (-45, -114)
  line L535 (-64.3301, -107.8397) -> (-62.0096, -106.5)
  line L536 (-32, -64) -> (-38.3975, -64)
  line L537 (-35.6699, -78.1987) -> (-40, -80.6987)
  line L538 (-25.6699, -60.8782) -> (-30, -63.3782)
  line L539 (-29.3301, -64.5385) -> (-25, -62.0385)
  line L540 (-70, -122.6603) -> (-67.6795, -124)
  line L541 (-20.6699, -64.5385) -> (-20.6699, -69.5385)
  line L542 (-20.6699, -116.5) -> (-20.6699, -121.5)
  arc A172 (-28, -59) -> (-30, -61) centre (-28, -61) ccw
  arc A173 (-18.3454, -63.9699) -> (-18, -64) centre (-18, -62) ccw
  line L543 (-19.3301, -116.5) -> (-19.3301, -119.5064)
  line L544 (-30.6699, -64.5385) -> (-30.6699, -69.5385)
  line L545 (-75, -114) -> (-70.6699, -116.5)
  line L546 (-20, -61) -> (-20, -62)
  arc A174 (-32, -64) -> (-31.6546, -63.9699) centre (-32, -62) ccw
  line L547 (-19.3301, -69.5385) -> (-19.3301, -64.5385)
  arc A175 (-20, -62) -> (-19.6271, -63.163) centre (-18, -62) ccw
  line L548 (-19.3301, -64.5385) -> (-18.3454, -63.9699)
  line L549 (-24.3301, -59) -> (-22, -59)
  line L550 (-30, -62) -> (-30, -61)
  arc A176 (-17, -119) -> (-15, -117) centre (-17, -117) ccw
  line L551 (-25, -62.0385) -> (-20.6699, -64.5385)
  line L552 (-25.6699, -59) -> (-25.6699, -60.8782)
  line L553 (-70.6699, -121.5) -> (-75, -124)
  line L554 (-65.6699, -112.8398) -> (-70, -115.3397)
  line L555 (-10.6699, -69.5064) -> (-10.6699, -69.5385)
  line L556 (-17, -64) -> (-18, -64)
  line L557 (-20.6699, -121.5) -> (-25, -124)
  line L558 (-45, -89.359) -> (-49.3301, -86.859)
  line L559 (-25, -89.359) -> (-29.3301, -86.859)
  line L560 (-57.9904, -106.5) -> (-55.6699, -107.8398)
  line L561 (-138.0873, -103) -> (-139.3301, -103)
  line L562 (-11.9128, -103) -> (-10.6699, -103)
  arc A177 (-125.7732, -114.9644) -> (-126.72, -114.993) centre (-126.22, -115.8591) ccw
  line L563 (-1, 108) -> (-1, 90)
  line L564 (-1, 42) -> (-1, 60)
  line L565 (-197, 42) -> (-197, 60)
  line L566 (-35, -54) -> (-35, -49)
  line L567 (-15, -49) -> (-15, -54)
  line L568 (-30, -49) -> (-20, -49)
  line L569 (-20, -49) -> (-20, -54)
  line L570 (-20, -54) -> (-30, -54)
  line L571 (-30, -54) -> (-30, -49)
  line L572 (-120.0001, -54) -> (-120.0001, -49)
  line L573 (-120.0001, -49) -> (-130.0001, -49)
  line L574 (-120.0001, -54) -> (-130.0001, -54)
  line L575 (-130.0001, -49) -> (-130.0001, -54)
  line L576 (15, -50) -> (15, -50)
  line L577 (15, -50) -> (10, -50)
  line L578 (10, -50) -> (10, -45)
  line L579 (5, -40) -> (5, -40)
  line L580 (0, -45) -> (0, -50)
  line L581 (0, -50) -> (-5, -50)
  line L582 (-5, -50) -> (-5, -50)
  arc A178 (-5, -50) -> (-1.4897, -54.7729) centre (0, -50) ccw
  arc A179 (11.4897, -54.7729) -> (15, -50) centre (10, -50) ccw
  arc A180 (5, -40) -> (0, -45) centre (5, -45) ccw
  arc A181 (10, -45) -> (5, -40) centre (5, -45) ccw
  line L583 (-13.9289, 15) -> (-54, 15)
  line L584 (-457, 135) -> (-447, 135)
  line L585 (-447, 115) -> (-452, 115)
  line L586 (-452, 35) -> (-457, 35)
  line L587 (-457, 35) -> (-457, 35)
  arc A182 (-457, 35) -> (-462, 30) centre (-457, 30) ccw
  line L588 (-462, 20) -> (-462, 30)
  arc A183 (-462, 20) -> (-457, 15) centre (-457, 20) ccw
  line L589 (-457, 15) -> (-447, 15)
  line L590 (-457, 30) -> (-452, 30)
  line L591 (-457, 20) -> (-452, 20)
  line L592 (-452, 35) -> (-447, 35)
  line L593 (-457, 30) -> (-457, 20)
  line L594 (95, 134.9866) -> (99.9997, 134.9859)
  line L595 (100.0021, 134.9863) -> (99.9997, 134.9859)
  arc A184 (105.0018, 129.986) -> (100.0021, 134.9863) centre (100.0018, 129.9863) ccw
  line L596 (105.0016, 119.999) -> (105.0018, 129.986)
  arc A185 (100.0016, 114.999) -> (105.0016, 119.999) centre (100.0016, 119.999) ccw
  line L597 (100.0018, 129.9863) -> (95.0022, 129.9866)
  line L598 (100.0016, 119.999) -> (95.0018, 119.9993)
  line L599 (100.0018, 129.9863) -> (100.0016, 119.999)
  line L600 (90, 134.9873) -> (95, 134.9866)
  line L601 (100.0021, 15.0137) -> (99.9997, 15.0141)
  arc A186 (100.0021, 15.0137) -> (105.0018, 20.014) centre (100.0018, 20.0137) ccw
  line L602 (105.0016, 30.001) -> (105.0018, 20.014)
  arc A187 (105.0016, 30.001) -> (100.0016, 35.001) centre (100.0016, 30.001) ccw
  line L603 (100.0016, 35.001) -> (90, 35.0009)
  line L604 (90, 134.9873) -> (90, 145)
  line L605 (90, 90) -> (90, 115)
  line L606 (90, 115) -> (100.0016, 114.999)
  line L607 (90, 5) -> (90, 15)
  line L608 (90, 15) -> (99.9997, 15.0141)
  line L609 (95.0019, 122.4929) -> (80.0019, 122.4936)
  line L610 (80.0019, 122.4936) -> (80.002, 124.9936)
  line L611 (95.0021, 127.4929) -> (80.0021, 127.4936)
  line L612 (80.0021, 127.4936) -> (80.002, 124.9936)
  line L613 (95.0022, 129.9866) -> (95.0021, 127.4929)
  line L614 (95.0019, 122.4929) -> (95.0018, 119.9993)
  line L615 (100.0018, 20.0137) -> (100.0016, 30.001)
  line L616 (95.0022, 20.0134) -> (95.0021, 22.5071)
  line L617 (95.0021, 22.5071) -> (80.0021, 22.5064)
  line L618 (80.0021, 22.5064) -> (80.002, 25.0064)
  line L619 (100.0018, 20.0137) -> (95.0022, 20.0134)
  line L620 (95.0019, 27.5071) -> (95.0018, 30.0007)
  line L621 (95.0019, 27.5071) -> (80.0019, 27.5064)
  line L622 (80.0019, 27.5064) -> (80.002, 25.0064)
  line L623 (100.0016, 30.001) -> (95.0018, 30.0007)
  line L624 (-452, 27.5) -> (-437, 27.5)
  line L625 (-437, 27.5) -> (-437, 25)
  line L626 (-452, 22.5) -> (-437, 22.5)
  line L627 (-437, 22.5) -> (-437, 25)
  line L628 (-452, 30) -> (-452, 27.5)
  line L629 (-452, 22.5) -> (-452, 20)
  line L630 (-457, 130) -> (-452, 130)
  line L631 (-452, 127.5) -> (-452, 130)
  line L632 (-437, 127.5) -> (-437, 125)
  line L633 (-452, 127.5) -> (-437, 127.5)
  line L634 (-452, 120) -> (-452, 122.5)
  line L635 (-452, 122.5) -> (-437, 122.5)
  line L636 (-437, 122.5) -> (-437, 125)
  line L637 (-457, 120) -> (-452, 120)
  line L638 (-457, 120) -> (-457, 130)
  circle A188 centre (-432, 95) radius 1.5
  circle A189 centre (-392, 135) radius 1.5
  line L639 (5, -50) -> (2.5, -50)
  line L640 (2.5, -50) -> (2.5, -45)
  line L641 (2.5, -45) -> (7.5, -45)
  line L642 (7.5, -45) -> (7.5, -50)
  line L643 (7.5, -50) -> (5, -50)
  line L644 (25, -50) -> (25, -50)
  line L645 (30, -45) -> (30, -40)
  line L646 (30, -40) -> (33, -40)
  line L647 (35, -38) -> (35, -37)
  line L648 (33, -35) -> (27, -35)
  line L649 (25, -37) -> (25, -48.873)
  arc A190 (26.25, -49.8412) -> (30, -45) centre (25, -45) ccw
  arc A191 (33, -40) -> (35, -38) centre (33, -38) ccw
  arc A192 (35, -37) -> (33, -35) centre (33, -37) ccw
  arc A193 (27, -35) -> (25, -37) centre (27, -37) ccw
  circle A194 centre (-408, 61) radius 1
  circle A195 centre (-380, 89) radius 1
  arc A196 (-384.7916, 87.5714) -> (-381.4286, 84.2084) centre (-380, 89) ccw
  arc A197 (-403.2084, 62.4286) -> (-401.2918, 61) centre (-401.2918, 63) ccw
  arc A198 (-408, 67.7082) -> (-406.5714, 65.7916) centre (-406, 67.7082) ccw
  arc A199 (-380, 82.2918) -> (-381.4286, 84.2084) centre (-382, 82.2918) ccw
  arc A200 (-384.7916, 87.5714) -> (-386.7082, 89) centre (-386.7082, 87) ccw
  arc A201 (25, -48.873) -> (26.25, -49.8412) centre (26, -48.873) ccw
  line L650 (-315, -19.9102) -> (-319, -19.9102)
  arc A202 (-323, -15.9098) -> (-319, -19.9102) centre (-319, -15.9102) ccw
  arc A203 (-315, -19.9102) -> (-311, -15.9102) centre (-315, -15.9102) ccw
  arc A204 (-358, 30.9999) -> (-362, 27) centre (-358, 26.9999) ccw
  line L651 (-362, 27) -> (-362, 23)
  arc A205 (-362, 23) -> (-358, 18.9999) centre (-358, 22.9999) ccw
  arc A206 (-330, 43) -> (-332, 41) centre (-330, 41) ccw
  line L652 (-332, 41) -> (-332, 37)
  arc A207 (-334, 35) -> (-332, 37) centre (-334, 37) ccw
  line L653 (-337, 35) -> (-334, 35)
  line L654 (-332, 15) -> (-337, 15)
  line L655 (-332, 23.9999) -> (-332, 15)
  arc A208 (-330, 25.9999) -> (-332, 23.9999) centre (-330, 23.9999) ccw
  line L656 (-267, 26) -> (-330, 25.9999)
  line L657 (-283, 53) -> (-267, 53)
  line L658 (-330, 43) -> (-287, 43)
  line L659 (-285, 45) -> (-285, 51)
  arc A209 (-287, 43) -> (-285, 45) centre (-287, 45) ccw
  arc A210 (-283, 53) -> (-285, 51) centre (-283, 51) ccw
  line L660 (-128, 15) -> (-108, 15)
  line L661 (-128, 135) -> (-108, 135)
  line L662 (-429, 90) -> (-440, 90)
  line L663 (-444, 86) -> (-444, 64)
  line L664 (-440, 60) -> (-429, 60)
  line L665 (-425, 64) -> (-425, 86)
  arc A211 (-440, 90) -> (-444, 86) centre (-440, 86) ccw
  arc A212 (-425, 86) -> (-429, 90) centre (-429, 86) ccw
  arc A213 (-429, 60) -> (-425, 64) centre (-429, 64) ccw
  arc A214 (-444, 64) -> (-440, 60) centre (-440, 64) ccw
  line L666 (-64.5, 72.5) -> (-85.6381, 72.5)
  line L667 (-96.3619, 72.5) -> (-97, 72.5)
  arc A215 (-62.2143, 48.8299) -> (-62.2143, 41.1701) centre (-59, 45) ccw
  arc A216 (-55.7857, 41.1701) -> (-55.7857, 48.8299) centre (-59, 45) ccw
  line L668 (-61.5, 69.5) -> (-61.5, 50.3619)
  line L669 (-61.5, 39.6381) -> (-61.5, 18)
  line L670 (-56.5, 17.5) -> (-56.5, 39.6381)
  line L671 (-56.5, 50.3619) -> (-56.5, 75)
  line L672 (-96.3619, 77.5) -> (-97, 77.5)
  arc A217 (-100, 80.5) -> (-97, 77.5) centre (-97, 80.5) ccw
  line L673 (-100, 132) -> (-100, 80.5)
  arc A218 (-97, 135) -> (-100, 132) centre (-97, 132) ccw
  line L674 (-64.5, 135) -> (-97, 135)
  arc A219 (-61.5, 132) -> (-64.5, 135) centre (-64.5, 132) ccw
  line L675 (-61.5, 110.3619) -> (-61.5, 132)
  arc A220 (-62.2143, 108.8299) -> (-62.2143, 101.1701) centre (-59, 105) ccw
  line L676 (-61.5, 80.5) -> (-61.5, 99.6381)
  arc A221 (-64.5, 77.5) -> (-61.5, 80.5) centre (-64.5, 80.5) ccw
  line L677 (-64.5, 77.5) -> (-85.6381, 77.5)
  arc A222 (-94.8299, 71.7857) -> (-87.1701, 71.7857) centre (-91, 75) ccw
  arc A223 (-87.1701, 78.2143) -> (-94.8299, 78.2143) centre (-91, 75) ccw
  arc A224 (-94.8299, 71.7857) -> (-96.3619, 72.5) centre (-96.3619, 70.5) ccw
  arc A225 (-96.3619, 77.5) -> (-94.8299, 78.2143) centre (-96.3619, 79.5) ccw
  arc A226 (-87.1701, 78.2143) -> (-85.6381, 77.5) centre (-85.6381, 79.5) ccw
  arc A227 (-85.6381, 72.5) -> (-87.1701, 71.7857) centre (-85.6381, 70.5) ccw
  arc A228 (-61.5, 99.6381) -> (-62.2143, 101.1701) centre (-63.5, 99.6381) ccw
  arc A229 (-62.2143, 108.8299) -> (-61.5, 110.3619) centre (-63.5, 110.3619) ccw
  arc A230 (-62.2143, 48.8299) -> (-61.5, 50.3619) centre (-63.5, 50.3619) ccw
  arc A231 (-61.5, 39.6381) -> (-62.2143, 41.1701) centre (-63.5, 39.6381) ccw
  arc A232 (-55.7857, 41.1701) -> (-56.5, 39.6381) centre (-54.5, 39.6381) ccw
  arc A233 (-56.5, 50.3619) -> (-55.7857, 48.8299) centre (-54.5, 50.3619) ccw
  line L678 (-11, 132.5) -> (-11, 75)
  arc A234 (-11, 132.5) -> (-13.5, 135) centre (-13.5, 132.5) ccw
  line L679 (-13.9289, 135) -> (-13.5, 135)
  line L680 (-13.9289, 135) -> (-54, 135)
  arc A235 (-54, 135) -> (-56.5, 132.5) centre (-54, 132.5) ccw
  line L681 (-56.5, 132.5) -> (-56.5, 110.3619)
  arc A236 (-56.5, 110.3619) -> (-55.7857, 108.8299) centre (-54.5, 110.3619) ccw
  arc A237 (-55.7857, 101.1701) -> (-55.7857, 108.8299) centre (-59, 105) ccw
  arc A238 (-55.7857, 101.1701) -> (-56.5, 99.6381) centre (-54.5, 99.6381) ccw
  line L682 (-56.5, 99.6381) -> (-56.5, 75)
  circle A239 centre (-59, 105) radius 1.5
  arc A240 (1.9074, -58.4876) -> (1.899, -58.4495) centre (-5, -60) ccw
  arc A241 (8.101, -58.4495) -> (8.0926, -58.4876) centre (15, -60) ccw
  arc A242 (0.4822, -67.1423) -> (9.5178, -67.1423) centre (5, -65) ccw
  arc A243 (1.899, -58.4495) -> (-1.4897, -54.7729) centre (-2.9793, -59.5459) ccw
  arc A244 (11.4897, -54.7729) -> (8.101, -58.4495) centre (12.9793, -59.5459) ccw
  circle A245 centre (5, -65) radius 2
  arc A246 (1.1111, -61.8573) -> (8.8889, -61.8573) centre (5, -65) ccw
  arc A247 (1.1111, -61.8573) -> (1.9074, -58.4876) centre (-2, -59.3431) ccw
  arc A248 (8.0926, -58.4876) -> (8.8889, -61.8573) centre (12, -59.3431) ccw
  line L683 (-323, -15.9098) -> (-322.9979, 2.9998)
  line L684 (-311, -15.9102) -> (-311, 3)
  line L685 (-327, 5) -> (-324.9979, 5)
  line L686 (-309, 5) -> (-307, 5)
  arc A249 (-322.9979, 2.9998) -> (-324.9979, 5) centre (-324.9979, 3) ccw
  arc A250 (-309, 5) -> (-311, 3) centre (-309, 3) ccw
  line L687 (-337, 15) -> (-337, 16.9999)
  line L688 (-337, 33) -> (-337, 35)
  arc A251 (-339, 31) -> (-337, 33) centre (-339, 33) ccw
  arc A252 (-337, 16.9999) -> (-339, 18.9999) centre (-339, 16.9999) ccw
  line L689 (-267, 26) -> (-204, 25.9999)
  arc A253 (-202, 23.9999) -> (-204, 25.9999) centre (-204, 23.9999) ccw
  line L690 (-202, 23.9999) -> (-202, 15)
  line L691 (-202, 15) -> (-197, 15)
  line L692 (-197, 15) -> (-197, 16.9999)
  arc A254 (-195, 18.9999) -> (-197, 16.9999) centre (-195, 16.9999) ccw
  arc A255 (-176, 18.9999) -> (-172, 23) centre (-176, 22.9999) ccw
  line L693 (-172, 27) -> (-172, 23)
  arc A256 (-172, 27) -> (-176, 30.9999) centre (-176, 26.9999) ccw
  arc A257 (-197, 33) -> (-195, 31) centre (-195, 33) ccw
  line L694 (-197, 33) -> (-197, 35)
  line L695 (-197, 35) -> (-200, 35)
  arc A258 (-202, 37) -> (-200, 35) centre (-200, 37) ccw
  line L696 (-202, 41) -> (-202, 37)
  arc A259 (-202, 41) -> (-204, 43) centre (-204, 41) ccw
  line L697 (-204, 43) -> (-241, 43)